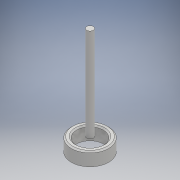
# Autodesk Inventor part: Part3
Saved by Autodesk Inventor 2017 (Build 210142000, 142)
## iProperties
Part Number: Part3
Material: 一般
Document SubType Name: Modeling
Designer: 7989303491
Density: 1 g/cm^3
Appearance: 既定
Author: 7989303491
Autodesk Inventor part; units mm, degrees
ref_plane "YZ Plane" through (0, 0, 0) normal (1, 0, 0) x (0, 1, 0)
ref_plane "XZ Plane" through (0, 0, 0) normal (0, 1, 0) x (-1, 0, 0)
ref_plane "XY Plane" through (0, 0, 0) normal (0, 0, 1) x (1, 0, 0)
sketch "スケッチ1" plane through (0, 0, 0) normal (0, 0, 1) x (1, 0, 0)
  circle A0 centre (0, 0) radius 10
  circle A1 centre (0, 0) radius 13.9508
  dimension "d0" = 20
  constraints: 2 centre point, 2 coincident
  measures "d0" diameter of A0
extrude "押し出し1" add sketch "スケッチ1" along normal blind 10
chamfer "面取り1" distance 1 angle 45 1 edges at (-13.9508, 0, 10)
chamfer "面取り2" distance 1 angle 45 1 edges at (-10, 0, 10)
sketch "スケッチ2" plane through (0, 0, 10) normal (0, 0, 1) x (1, 0, 0)
  circle A0 centre (0, 0) radius 2.5
  dimension "d9" = 5
  constraints: 1 centre point, 1 coincident
  measures "d9" diameter of A0
extrude "押し出し2" add sketch "スケッチ2" along normal blind 70
